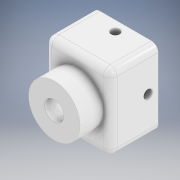
# Autodesk Inventor part: Case_Holder
Saved by Autodesk Inventor 2020 (Build 240168000, 168)
## iProperties
Created: 2020-02-24
Part Number: Case_Holder
Material: 일반
Document SubType Name: Modeling
Designer: Knowblesse
Density: 1 g/cm^3
Appearance: 기본값
Author: Knowblesse
## iProperties of the stored document _3D 인쇄.ipt
Created: 2020-04-09
Part Number: _3D 인쇄
Material: 일반
Document SubType Name: Modeling
Designer: Knowblesse
Density: 1 g/cm^3
Appearance: 기본값
Author: Knowblesse
Autodesk Inventor part; units mm, degrees
ref_plane "YZ Plane" through (0, 0, 0) normal (1, 0, 0) x (0, 1, 0)
ref_plane "XZ Plane" through (0, 0, 0) normal (0, 1, 0) x (-1, 0, 0)
ref_plane "XY Plane" through (0, 0, 0) normal (0, 0, 1) x (1, 0, 0)
sketch "스케치1" plane through (0, 0, 0) normal (0, 0, 1) x (1, 0, 0)
  line L0 (0, 0) -> (13, 0)
  line L1 (13, 0) -> (13, 16)
  line L2 (13, 16) -> (0, 16)
  line L3 (0, 16) -> (0, 0)
  line L4 (-3, 19) -> (16, 19)
  line L5 (16, 19) -> (16, -3)
  line L6 (16, -3) -> (-3, -3)
  line L7 (-3, -3) -> (-3, 19)
  dimension "d0" = 13
  dimension "d1" = 16
  dimension "d2" = 3
  constraints: 16 end point, 4 parallel, 2 perpendicular, 1 horizontal, 3 other
  measures "d0" distance of L1.end L2.end
  measures "d1" distance between parallel lines of L0 L2
  measures "d2" distance between parallel lines of L2 L4
extrude "돌출1" add sketch "스케치1" along normal blind 7
sketch "스케치2" plane through (0, 0, 7) normal (0, 0, 1) x (1, 0, 0)
  line L0 (-3, 19) -> (-3, -3) projected
  line L1 (-3, -3) -> (16, -3) projected
  line L2 (16, -3) -> (16, 19) projected
  line L3 (16, 19) -> (-3, 19) projected
  line L4 (13, 0) -> (0, 0) projected
  line L5 (0, 0) -> (0, 16) projected
  line L6 (0, 16) -> (13, 16) projected
  line L7 (13, 16) -> (13, 0) projected
  line L8 (1, 16) -> (1, 0)
  line L9 (13, 0) -> (0, 0) projected
  line L10 (12, 16) -> (12, 0)
  line L11 (0, 16) -> (13, 16) projected
  dimension "d5" = 1
  dimension "d6" = 1
  constraints: 4 end point, 4 point on line, 2 perpendicular
  measures "d5" distance between parallel lines of L5 L8
  measures "d6" distance between parallel lines of L7 L10
extrude "돌출2" add sketch "스케치2" along normal blind 6 contours L3 L2 L1 L0 | L4 L10 L6 L7 | L4 L5 L6 L8
fillet "모깎기1" radius 2 4 edges at (0, 16, 3.5) (13, 16, 3.5) (13, 0, 3.5) (0, 0, 3.5)
sketch "스케치3" plane through (0, 0, 13) normal (0, 0, 1) x (1, 0, 0)
  line L0 (-3, -3) -> (16, -3) projected
  line L1 (16, -3) -> (16, 19) projected
  line L2 (16, 19) -> (-3, 19) projected
  line L3 (-3, 19) -> (-3, -3) projected
  line L4 (11, 0) -> (2, 0) projected
  arc A0 (1, 0.2679) -> (2, 0) centre (2, 2) ccw projected
  line L5 (1, 0.2679) -> (1, 15.7321) projected
  arc A1 (2, 16) -> (1, 15.7321) centre (2, 14) ccw projected
  line L6 (2, 16) -> (11, 16) projected
  arc A2 (12, 15.7321) -> (11, 16) centre (11, 14) ccw projected
  line L7 (12, 15.7321) -> (12, 0.2679) projected
  arc A3 (11, 0) -> (12, 0.2679) centre (11, 2) ccw projected
  point P0 (0, 0)
extrude "돌출3" add sketch "스케치3" along normal blind 1 contours L3 L2 L1 L0 | L4 A0 L5 A1 L6 A2 L7 A3
fillet "모깎기2" radius 2 8 edges at (16, -3, 7) (-3, -3, 7) (16, 19, 7) (-3, 19, 7) (16, 8, 14) (6.5, -3, 14) (-3, 8, 14) (6.5, 19, 14)
sketch "스케치5" plane through (0, 0, 7) normal (0, 0, -1) x (-1, 0, 0)
  arc A0 (-1, 0.2679) -> (0, 2) centre (-2, 2) ccw projected
  line L0 (0, 2) -> (0, 14) projected
  arc A1 (0, 14) -> (-1, 15.7321) centre (-2, 14) ccw projected
  line L1 (-1, 0.2679) -> (-1, 15.7321) projected
  point P0 (0, 0)
extrude "돌출4" add sketch "스케치5" along normal blind 1.5
sketch "스케치6" plane through (0, 0, 14) normal (0, 0, 1) x (1, 0, 0)
  line L0 (-1, 17) -> (14, 17) projected
  line L1 (-1, -1) -> (-1, 17) projected
  line L2 (14, -1) -> (-1, -1) projected
  line L3 (14, 17) -> (14, -1) projected
  point P0 (0, 0)
  point P1 (6.5, 8)
  point P2 (6.5, -1)
  point P3 (14, 8)
  constraints: 2 midpoint, 1 horizontal alignment, 1 vertical alignment
hole "구멍2" at (6.5, 8, 14) direction (0, 0, -1) diameter 3 end through all
sketch "스케치7" plane through (0, 0, 14) normal (0, 0, 1) x (1, 0, 0)
  circle A0 centre (6.5, 8) radius 1.5 projected
  line L0 (-1, 17) -> (14, 17) projected
  line L1 (-1, -1) -> (-1, 17) projected
  line L2 (14, -1) -> (-1, -1) projected
  line L3 (14, 17) -> (14, -1) projected
  circle A1 centre (6.5, 8) radius 2.8
  circle A2 centre (6.5, 8) radius 1.5 projected
  circle A3 centre (6.5, 8) radius 7.5
  point P0 (0, 0)
  dimension "d32" = 5.6
  constraints: 2 centre point, 2 coincident, 1 tangent
  measures "d32" diameter of A1
extrude "돌출5" add sketch "스케치7" along normal blind 6.8 contours A3
sketch "스케치8" plane through (16, -1, 0) normal (1, 0, 0) x (0, 0, -1)
  line L0 (-12, 18) -> (0, 18) projected
  line L1 (-12, 0) -> (-12, 18) projected
  line L2 (0, 0) -> (-12, 0) projected
  line L3 (0, 0) -> (0, 18) projected
  point P0 (0, 1)
  point P1 (-3, 9)
  point P2 (-12, 9)
  dimension "d35" = 3
  constraints: 1 horizontal alignment, 1 midpoint
  measures "d35" distance from line of point (-3, 9) L3
hole "구멍3" at (16, 8, 3) direction (-1, 0, 0) diameter 2.5 end through all
sketch "스케치9" plane through (-1, 19, 0) normal (0, 1, 0) x (1, 0, 0)
  line L0 (0, -12) -> (0, 0) projected
  line L1 (15, -12) -> (0, -12) projected
  line L2 (15, 0) -> (15, -12) projected
  line L3 (15, 0) -> (0, 0) projected
  point P0 (1, 0)
  point P1 (7.5, -3)
  point P2 (7.5, -12)
  dimension "d43" = 3
  constraints: 1 midpoint, 1 vertical alignment
  measures "d43" distance from line of point (7.5, -3) L3
hole "구멍4" at (6.5, 19, 3) direction (0, -1, 0) diameter 2.5 end through all
